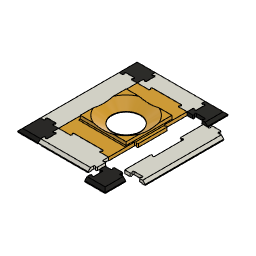
JarBase v9 (Autodesk Fusion 360 design; units mm, degrees)
Autodesk Fusion 360 part; units mm, degrees
sketch "Sketch1" plane through (0, 0, 0) normal (0, 0, 1) x (1, 0, 0) in component "JarBase"
  line L0 (32.5, -50) -> (-32.5, -50)
  line L1 (-32.5, -50) -> (-32.5, 50)
  line L2 (-32.5, 50) -> (32.5, 50)
  line L3 (32.5, 50) -> (32.5, -50)
  line L4 (32.5, -50) -> (-32.5, 50) construction
  line L5 (-32.5, -50) -> (32.5, 50) construction
  line L6 (28.5, -30) -> (-28.5, -30)
  line L7 (-28.5, -30) -> (-28.5, 30)
  line L8 (-28.5, 30) -> (28.5, 30)
  line L9 (28.5, 30) -> (28.5, -30)
  line L10 (28.5, -30) -> (-28.5, 30) construction
  line L11 (-28.5, -30) -> (28.5, 30) construction
  line L12 (28.5, 46) -> (-28.5, 46)
  line L13 (-28.5, 46) -> (-28.5, -46)
  line L14 (-28.5, -46) -> (28.5, -46)
  line L15 (28.5, -46) -> (28.5, 46)
  line L16 (28.5, 46) -> (-28.5, -46) construction
  line L17 (-28.5, 46) -> (28.5, -46) construction
  line L18 (-20, -46) -> (-16, -50)
  line L19 (-20, -46) -> (-14.5795, -46) construction
  line L20 (20, -46) -> (16, -50)
  line L21 (20, -46) -> (25.374, -46) construction
  line L22 (28.5, 16) -> (32.5, 20)
  line L23 (28.5, 16) -> (37.0214, 16) construction
  line L24 (28.5, -16) -> (32.5, -20)
  line L25 (28.5, -16) -> (34.342, -16) construction
  line L26 (-28.5, 46) -> (-32.5, 46)
  line L27 (16, 46) -> (20, 50)
  line L28 (16, 46) -> (23.4683, 46) construction
  line L29 (-16.4731, 46) -> (-20, 50)
  line L30 (-19.9118, 49.9) -> (19.9, 49.9)
  line L31 (15.8586, 46) -> (19.7586, 49.9)
  line L32 (-16.3398, 46) -> (-19.8667, 50)
  line L33 (28.5, 15.8586) -> (32.5, 19.8586)
  line L34 (32.4, 19.9) -> (32.4, -19.9)
  line L35 (32.5, -19.8586) -> (28.5, -15.8586)
  line L36 (28.5, -46) -> (28.5, -50)
  circle A0 centre (0, 0) radius 16.5
  line L37 (-55.4758, 0) -> (62.2812, 0) construction
  line L38 (-28.5, -20) -> (-32.5, -16)
  line L39 (-28.5, -20) -> (-22.6366, -20) construction
  line L40 (-28.5, 20) -> (-32.5, 16)
  line L41 (-28.5, 20) -> (-23.3061, 20) construction
  line L42 (0, 81.2463) -> (0, -111.1195) construction
  circle A1 centre (0, 0) radius 17.5
  dimension "d3" = 65
  dimension "d4" = 100
  dimension "d7" = 57
  dimension "d8" = 60
  dimension "d13" = 57
  dimension "d14" = 92
  dimension "d26" = 40
  dimension "d27" = 45
  dimension "d28" = 135
  dimension "d33" = 45
  dimension "d34" = 45
  dimension "d35" = 40
  dimension "d40" = 45
  dimension "d42" = 40
  dimension "d43" = 0.1
  dimension "d44" = 0.1
  dimension "d45" = 0.1
  dimension "d46" = 0.1
  dimension "d47" = 0.1
  dimension "d48" = 0.1
  dimension "d57" = 33
  dimension "d58" = 135
  dimension "d59" = 135
  dimension "d60" = 40
  dimension "d217" = 35
  constraint horizontal L0
  constraint perpendicular L0 L1
  constraint parallel L0 L2
  constraint parallel L1 L3
  constraint coincident L4 A0.centre
  constraint coincident L5 A0.centre
  constraint coincident A0.centre A1.centre
  constraint horizontal L6
  constraint perpendicular L6 L7
  constraint parallel L6 L8
  constraint parallel L7 L9
  constraint coincident L10 A0.centre
  constraint coincident L11 A0.centre
  constraint horizontal L12
  constraint perpendicular L12 L13
  constraint parallel L12 L14
  constraint parallel L13 L15
  constraint coincident L16 A0.centre
  constraint coincident L17 A0.centre
  constraint horizontal L19
  constraint horizontal L21
  constraint coincident L0 L20.end
  constraint horizontal L23
  constraint horizontal L25
  constraint coincident L3 L24.end
  constraint coincident L1 L26.end
  constraint perpendicular L1 L26
  constraint horizontal L28
  constraint coincident L2 L27.end
  constraint coincident L2 L29.end
  constraint coincident L14 L20.start
  constraint coincident L15 L24.start
  constraint coincident L15 L22.start
  constraint coincident L12 L27.start
  constraint coincident L12 L29.start
  constraint coincident L29 L30.start
  constraint coincident L27 L30.end
  constraint parallel L2 L30
  constraint coincident L12 L31.start
  constraint coincident L30 L31.end
  constraint parallel L27 L31
  constraint coincident L12 L32.start
  constraint coincident L2 L32.end
  constraint parallel L29 L32
  constraint coincident L15 L33.start
  constraint coincident L3 L33.end
  constraint parallel L22 L33
  constraint coincident L22 L34.start
  constraint coincident L24 L34.end
  constraint vertical L34
  constraint coincident L3 L35.start
  constraint coincident L15 L35.end
  constraint parallel L24 L35
  constraint coincident L0 L36.end
  constraint perpendicular L0 L36
  constraint coincident L0 L18.end
  constraint horizontal L37
  constraint coincident A0.centre L37
  constraint horizontal L39
  constraint coincident L1 L38.end
  constraint horizontal L41
  constraint coincident L7 L40.start
  constraint coincident L1 L40.end
  constraint symmetric L38.start L37 L40.start
  constraint coincident L3 L22.end
  constraint symmetric L22.end L24.end L37
  constraint coincident L14 L18.start
  constraint perpendicular L14 L42
  constraint coincident A0.centre L42
  constraint symmetric L18.start L20.start L42
  constraint symmetric L27.end L29.end L42
  constraint concentric A0 A1
  measures "d3" distance of L1.end L2.end
  measures "d4" distance of L0 L2
  measures "d7" distance of L7.end L8.end
  measures "d8" distance of L6.end L7.end
  measures "d13" distance of L13.end L14.end
  measures "d14" distance of L12.end L13.end
  measures "d26" distance of L18.start L20.start
  measures "d27" angle of L18 L19
  measures "d28" angle of L20 L21
  measures "d33" angle of L22 L23
  measures "d34" angle of L24 L25
  measures "d35" vertical distance of L22.end L24.end
  measures "d40" angle of L27 L28
  measures "d42" distance of L27.end L29.end
  measures "d43" distance of L2 L30
  measures "d44" distance of L27 L31
  measures "d45" distance of L29 L32
  measures "d46" distance of L22 L33
  measures "d47" distance of L3 L34
  measures "d48" distance of L24 L35
  measures "d57" diameter of A0
  measures "d58" angle of L38 L39
  measures "d59" angle of L40 L41
  measures "d60" distance of L38.start L40.start
  measures "d217" diameter of A1
extrude "Extrude1" add sketch "Sketch1" along normal blind 4 contours L0 L14 L20 L36 | L6 L13 L14 L15 | L0 L1 L7 L13 L14 L18 L38 | L6 L7 L8 L9 L13 L15 | L9 L15 L33 L34 L35 | L1 L7 L13 L26 L40 | L8 L12 L13 L15 | L12 L30 L31 L32 | A0 | A1 makes body 1 in component "JarBase"
sketch "Sketch5" plane through (0, 0, 4) normal (0, 0, 1) x (-1, 0, 0) in component "JarBase"
  line L0 (-28.5, -15.8586) -> (-28.5, -46)
  line L1 (-28.5, -46) -> (-15.8586, -46)
  line L2 (-15.8586, -46) -> (-19.7586, -49.9)
  line L3 (-19.7586, -49.9) -> (19.7785, -49.9)
  line L4 (19.7785, -49.9) -> (16.3398, -46)
  line L5 (16.3398, -46) -> (32.5, -46)
  line L6 (32.5, -46) -> (32.5, -16)
  line L7 (32.5, 50) -> (16, 50)
  line L8 (16, 50) -> (20, 46)
  line L9 (20, 46) -> (-20, 46)
  line L10 (-28.5, 15.8586) -> (-32.4, 19.7586)
  line L11 (-32.4, 19.7586) -> (-32.4, -19.7586)
  line L12 (-32.4, -19.7586) -> (-28.5, -15.8586)
  line L13 (28, -28) -> (-28, -28)
  line L14 (-28, -28) -> (-28, 28)
  line L15 (-28, 28) -> (28, 28)
  line L16 (28, 28) -> (28, -28)
  line L17 (28, -28) -> (-28, 28) construction
  line L18 (-28, -28) -> (28, 28) construction
  line L19 (32.5, -16) -> (28.5, -20)
  line L20 (28.5, -20) -> (28.5, 20)
  line L21 (28.5, 20) -> (32.5, 16)
  line L22 (32.5, 16) -> (32.5, 50)
  line L23 (-20, 46) -> (-16, 50)
  line L24 (-16, 50) -> (-28.5, 50)
  line L25 (-28.5, 50) -> (-28.5, 15.8586)
  dimension "d51" = 56
  dimension "d52" = 56
  constraint horizontal L13
  constraint perpendicular L13 L14
  constraint parallel L13 L15
  constraint parallel L14 L16
  constraint coincident L17 origin
  constraint coincident L18 origin
  measures "d51" distance of L14.end L15.end
  measures "d52" distance of L13.end L14.end
extrude "Extrude3" add sketch "Sketch5" along normal blind 5 contours L13 L14 L15 L16 bodies 1 in component "JarBase"
sketch "Sketch3" plane through (0, 0, 9) normal (0, 0, 1) x (-1, 0, 0) in component "JarBase"
  circle A0 centre (0, 0) radius 30.5
  line L0 (30, 30) -> (-30, 30)
  line L1 (-30, 30) -> (-30, -30)
  line L2 (-30, -30) -> (30, -30)
  line L3 (30, -30) -> (30, 30)
  line L4 (28, 28) -> (-28, 28)
  line L5 (-28, 28) -> (-28, -28)
  line L6 (-28, -28) -> (28, -28)
  line L7 (28, -28) -> (28, 28)
  dimension "d12" = 61
  constraint coincident A0.centre origin
  measures "d12" diameter of A0
fillet "Fillet1" radius 1 16 edges at (-19.7785, 49.9, 2) (-16.3398, 46, 2) (19.7586, 49.9, 2) (15.8586, 46, 2) (32.4, 19.7586, 2) (32.4, -19.7586, 2) (28.5, -15.8586, 2) (28.5, 15.8586, 2) (20, -46, 2) (16, -50, 2) (-16, -50, 2) (-20, -46, 2) (-32.5, -16, 2) (-28.5, -20, 2) (-32.5, 16, 2) (-28.5, 20, 2) on bodies 1 in component "JarBase"
loft "Loft2" cut profiles "Sketch1", "Sketch3" section 1 contours A0 section 2 contours A0 L3 | A0 L3 L7 | A0 L4 L5 L6 L7 | A0 L0 L4 | A0 L0 | A0 L2 L6 | A0 L2 | A0 L1 L5 | A0 L1 bodies 1 in component "JarBase"
fillet "Fillet2" radius 1 4 edges at (0, 28, 4) (-28, 0, 4) (0, -28, 4) (28, 0, 4) on bodies 1 in component "JarBase"
sketch "Sketch1 (2)" plane through (0, 0, 0) normal (0, 0, 1) x (1, 0, 0) in component "TopEdge"
  line L0 (28.5, 46) -> (28.5, 71)
  line L1 (28.5, 71) -> (-32.5, 71)
  line L2 (-32.5, 71) -> (-32.5, 46)
  line L3 (-32.5, 52) -> (28.5, 52)
  line L4 (-32.5, 67) -> (28.5, 67)
  line L5 (-32.5, 50) -> (32.5, 50)
  line L6 (16, 46) -> (20, 50)
  line L7 (16, 46) -> (23.4683, 46)
  line L8 (28.5, 46) -> (-28.5, 46)
  line L9 (-16.4731, 46) -> (-20, 50)
  line L10 (-32.5, 46) -> (28.5, 46)
  line L11 (-20, 50) -> (-16.4731, 46)
  line L12 (20, 50) -> (16, 46)
  line L13 (20, 50) -> (-20, 50)
  line L14 (-28.5, 71) -> (-28.5, 46)
  line L15 (32.5, 66) -> (32.5, 51)
  line L16 (-32.5, 62) -> (-28.5, 66)
  line L17 (-32.5, 62) -> (-26.8431, 62) construction
  line L18 (-32.5, 55) -> (-28.5, 51)
  line L19 (-51.9513, 58.5) -> (44.591, 58.5) construction
  line L20 (32.5, 51) -> (28.5, 55)
  line L21 (32.5, 51) -> (38.1569, 51) construction
  line L22 (32.5, 66) -> (28.5, 62)
  line L23 (28.5, 61.8586) -> (32.4, 65.7586)
  line L24 (28.5, 55.1414) -> (32.5, 51.1414)
  line L25 (32.4, 65.7586) -> (32.4, 51.2414)
  point P0 (-32.5, 46)
  dimension "d62" = 15
  dimension "d63" = 4
  dimension "d64" = 25
  dimension "d81" = 4
  dimension "d82" = 4
  dimension "d83" = 45
  dimension "d84" = 90
  dimension "d85" = 15
  dimension "d86" = 135
  dimension "d87" = 90
  dimension "d88" = 15
  dimension "d89" = 0.1
  dimension "d90" = 0.1
  dimension "d91" = 0.1
  constraint vertical L0
  constraint horizontal L1
  constraint vertical L2
  constraint coincident L2 L3.start
  constraint coincident L0 L3.end
  constraint perpendicular L0 L3
  constraint coincident L2 L4.start
  constraint coincident L0 L4.end
  constraint perpendicular L0 L4
  constraint coincident L0.start L8.start
  constraint perpendicular L0 L10
  constraint coincident L9.end L11.start
  constraint coincident L9.start L11.end
  constraint coincident L6.end L12.start
  constraint coincident L6.start L7.start
  constraint coincident L0 L8.start
  constraint coincident L2 P0
  constraint coincident L1 L14.start
  constraint coincident L10 L8.end
  constraint perpendicular L10 L14
  constraint vertical L15
  constraint horizontal L17
  constraint coincident L2 L16.start
  constraint coincident L14 L16.end
  constraint coincident L2 L18.start
  constraint coincident L14 L18.end
  constraint horizontal L19
  constraint symmetric L1 L10 L19
  constraint symmetric L16.end L18.end L19
  constraint symmetric L15.start L15.end L19
  constraint horizontal L21
  constraint coincident L0 L20.end
  constraint coincident L0 L22.end
  constraint coincident L0 L23.start
  constraint parallel L22 L23
  constraint coincident L0 L24.start
  constraint coincident L15 L24.end
  constraint perpendicular L23 L24
  constraint coincident L23 L25.start
  constraint coincident L24 L25.end
  constraint parallel L15 L25
  constraint coincident L23.end L25
  measures "d62" distance of L3 L4
  measures "d63" distance of L1 L4
  measures "d64" distance of L1 L10
  measures "d81" distance of L2 L14
  measures "d82" distance of L0 L15
  measures "d83" angle of L16 L17
  measures "d84" angle of L16 L18
  measures "d85" distance of L16.end L18.end
  measures "d86" angle of L20 L21
  measures "d87" angle of L20 L22
  measures "d88" distance of L15.start L15.end
  measures "d89" distance of L22 L23
  measures "d90" distance of L20 L24
  measures "d91" distance of L15 L25
extrude "Extrude1'" add sketch "Sketch1 (2)" along normal blind 4 separate body contours L0 L3 L4 L14 | L0 L3 L5 L13 L14 | L0 L5 L6 L7 L8 L10 L12 | L0 L23 L24 L25 | L2 L3 L5 L14 L18 | L2 L3 L18 | L2 L4 L14 L16 | L5 L8 L9 L10 L11 L14 | L0 L1 L4 L14 | L1 L2 L4 L14 | L2 L5 L10 L14 makes body 2 in component "TopEdge"
fillet "Fillet1'" radius 1 4 edges at (-16.4731, 46, 2) (-20, 50, 2) (20, 50, 2) (16, 46, 2) on bodies 2 in component "TopEdge"
extrude "Extrude2" cut sketch "Sketch1 (2)" along normal blind 0.5 contours L0 L3 L4 L14 | L2 L3 L14 L16 L18 | L0 L23 L24 L25 | L2 L3 L18 | L2 L4 L14 L16 bodies 2 in component "TopEdge"
sketch "Sketch1 (3)" plane through (0, 0, 0) normal (0, 0, 1) x (1, 0, 0) in component "RIghtEdge"
  line L0 (28.5, 46) -> (53.5, 46)
  line L1 (53.5, 46) -> (53.5, -50)
  line L2 (53.5, -50) -> (28.5, -50)
  line L3 (28.5, -50) -> (28.5, 46)
  line L4 (28.5, 16) -> (32.5, 20)
  line L5 (32.5, 50) -> (32.5, -50)
  line L6 (28.5, -16) -> (32.5, -20)
  line L7 (28.5, 16) -> (32.5, 20)
  line L8 (32.5, -20) -> (28.5, -16)
  line L9 (32.5, 20) -> (32.5, -20)
  line L10 (49.5, 46) -> (49.5, -50)
  line L11 (34.5, 46) -> (34.5, -50)
  line L12 (41, 52.9761) -> (41, -53.7829) construction
  line L13 (29.9594, 46) -> (43.3433, 46) construction
  line L14 (48.5, 50) -> (44.5, 46)
  line L15 (48.5, 50) -> (48.5481, 50) construction
  line L16 (33.5, 50) -> (37.6148, 45.8852)
  line L17 (33.5, 50) -> (39.2756, 50) construction
  line L18 (33.5, 50) -> (48.5, 50)
  line L19 (33.6414, 50) -> (37.6414, 46)
  line L20 (48.3586, 50) -> (44.3586, 46)
  line L21 (33.7414, 49.9) -> (48.2586, 49.9)
  line L22 (33.5, -46) -> (48.5, -46)
  line L23 (48.5, -46) -> (44.5, -50)
  line L24 (48.5, -46) -> (54.0005, -46) construction
  line L25 (33.5, -46) -> (37.5, -50)
  point P0 (28.5, 46)
  dimension "d71" = 96
  dimension "d72" = 25
  dimension "d73" = 4
  dimension "d74" = 15
  dimension "d119" = 135
  dimension "d120" = 45
  dimension "d121" = 15
  dimension "d122" = 4
  dimension "d123" = 0.1
  dimension "d124" = 0.1
  dimension "d125" = 0.1
  dimension "d126" = 15
  dimension "d127" = 4
  dimension "d128" = 135
  dimension "d129" = 90
  constraint horizontal L0
  constraint vertical L1
  constraint horizontal L2
  constraint vertical L3
  constraint coincident P0 L0.start
  constraint coincident L4.start L7.start
  constraint coincident L4.end L7.end
  constraint coincident L6.end L8.start
  constraint coincident L6.start L8.end
  constraint coincident L0 L10.start
  constraint coincident L2 L10.end
  constraint perpendicular L2 L10
  constraint coincident L0 L11.start
  constraint coincident L2 L11.end
  constraint perpendicular L2 L11
  constraint perpendicular L0 L12
  constraint horizontal L13
  constraint coincident L0 L13.start
  constraint horizontal L15
  constraint horizontal L17
  constraint coincident L0 L14.end
  constraint symmetric L12 L14.start L16.start
  constraint coincident L18 L19.start
  constraint coincident L13 L19.end
  constraint coincident L18 L20.start
  constraint coincident L0 L20.end
  constraint perpendicular L19 L20
  constraint coincident L19 L21.start
  constraint coincident L20 L21.end
  constraint horizontal L21
  constraint parallel L16 L19
  constraint perpendicular L12 L22
  constraint horizontal L24
  constraint coincident L2 L23.end
  constraint coincident L2 L25.end
  constraint symmetric L12 L23 L25
  measures "d71" distance of L0.end L2
  measures "d72" distance of L1 L3
  measures "d73" distance of L1 L10
  measures "d74" distance of L10 L11
  measures "d119" angle of L14 L15
  measures "d120" angle of L16 L17
  measures "d121" distance of L14.start L16.start
  measures "d122" distance of L0 L18
  measures "d123" distance of L18 L21
  measures "d124" distance of L14 L20
  measures "d125" distance of L16 L19
  measures "d126" distance of L22.start L22.end
  measures "d127" distance of L2 L22
  measures "d128" angle of L23 L24
  measures "d129" angle of L23 L25
extrude "Extrude1''" add sketch "Sketch1 (3)" along normal blind 4 separate body contours L0 L19 L20 L21 | L0 L2 L10 L11 L22 L23 | L0 L2 L5 L9 L11 L22 L25 | L0 L1 L2 L10 | L0 L3 L4 L5 L7 | L2 L11 L25 | L2 L3 L5 L6 L8 makes body 3 in component "RIghtEdge"
extrude "Extrude2'" cut sketch "Sketch1 (3)" along normal blind 0.5 contours L0 L19 L20 L21 | L0 L2 L10 L11 L22 L23 | L2 L11 L22 L23 L25 | L2 L11 L25 bodies 3 in component "RIghtEdge"
fillet "Fillet1''" radius 1 4 edges at (28.5, 16, 2) (32.5, 20, 2) (28.5, -16, 2) (32.5, -20, 2) on bodies 3 in component "RIghtEdge"
fillet "Fillet2'" radius 1 4 edges at (-28.5, 66, 2.25) (-32.5, 62, 2.25) (-28.5, 51, 2) (-32.5, 55, 2.25) on bodies 2 in component "TopEdge"
fillet "Fillet3" radius 1 4 edges at (28.5, 61.8586, 2.25) (32.4, 65.7586, 2) (32.4, 51.2414, 2) (28.5, 55.1414, 2.25) on bodies 2 in component "TopEdge"
sketch "Sketch1 (4)" plane through (0, 0, 0) normal (0, 0, 1) x (1, 0, 0) in component "TopRightCorner"
  line L0 (32.5, 66) -> (28.5, 62)
  line L1 (32.5, 66) -> (32.5, 51)
  line L2 (32.5, 51) -> (28.5, 55)
  line L3 (28.5, 46) -> (28.5, 71)
  line L4 (28.5, 46) -> (53.5, 46)
  line L5 (28.5, 71) -> (53.5, 71)
  line L6 (53.5, 71) -> (53.5, 46)
  line L7 (53.5, 46) -> (28.5, 46)
  line L8 (28.5, 46) -> (28.5, 71)
  line L9 (32.5, 66) -> (28.5, 62)
  line L10 (28.5, 62) -> (28.5, 71)
  line L11 (32.5, 66) -> (32.5, 51)
  line L12 (32.5, 51) -> (28.5, 55)
  line L13 (28.5, 55) -> (28.5, 46)
  line L14 (28.5, 46) -> (37.5, 46)
  line L15 (44.5, 46) -> (53.5, 46)
  line L16 (33.5, 50) -> (48.5, 50)
  line L17 (33.5, 50) -> (37.6148, 45.8852)
  line L18 (48.5, 50) -> (44.5, 46)
  line L19 (53.5, 46) -> (44.3586, 46)
  line L20 (29.9594, 46) -> (43.3433, 46)
  line L21 (28.5, 46) -> (37.5, 46)
  line L22 (37.5, 46) -> (33.5, 50)
  line L23 (33.5, 50) -> (48.5, 50)
  line L24 (48.5, 50) -> (44.5, 46)
  line L25 (44.5, 46) -> (53.5, 46)
  point P0 (43.3433, 46)
  constraint horizontal L5
  constraint vertical L6
  constraint horizontal L7
  constraint vertical L8
  constraint coincident L4.end L6.end
  constraint coincident L3.end L5.start
  constraint coincident L0.start L1.start
  constraint coincident L0.end L9.end
  constraint coincident L1.end L2.start
  constraint coincident L2.end L12.end
  constraint coincident L3.start L4.start
  constraint parallel L20 L21
  constraint coincident L16.start L17.start
  constraint parallel L17 L22
  constraint coincident L16.end L18.start
  constraint parallel L18 L24
  constraint perpendicular L6 L25
extrude "Extrude1'''" add sketch "Sketch1 (4)" along normal blind 4 separate body contours L0 L1 L2 L3 L4 L5 L6 L7 L8 L9 L10 L11 L12 L13 L14 L15 L16 L17 L18 L19 L20 L21 L22 L23 L24 L25 makes body 4 in component "TopRightCorner"
fillet "Fillet1'''" radius 1 8 edges at (32.5, 51, 2) (28.5, 55, 2) (32.5, 66, 2) (28.5, 62, 2) (33.5, 50, 2) (37.5, 46, 2) (48.5, 50, 2) (44.5, 46, 2) on bodies 4 in component "TopRightCorner"
chamfer "Chamfer1" distance 3 angle 45 2 edges at (53.5, 58.5, 4) (41, 71, 4) on bodies 4 in component "TopRightCorner"
chamfer "Chamfer1'" distance 3 angle 45 1 edges at (53.5, -2, 4) on bodies 3 in component "RIghtEdge"
chamfer "Chamfer1''" distance 3 angle 45 1 edges at (-2, 71, 4) on bodies 2 in component "TopEdge"
fillet "Fillet3'" radius 1 8 edges at (37.6414, 46, 2.25) (33.7414, 49.9, 2.25) (48.2586, 49.9, 2.25) (44.3586, 46, 2.25) (37.5, -50, 2.25) (33.5, -46, 2) (48.5, -46, 2.25) (44.5, -50, 2.25) on bodies 3 in component "RIghtEdge"
sketch "Sketch1 (5)" plane through (0, 0, 0) normal (0, 0, 1) x (1, 0, 0) in component "BottomEdge"
  line L0 (32.5, -50) -> (-32.5, -50)
  line L1 (-20, -46) -> (-16, -50)
  line L2 (-28.5, -46) -> (28.5, -46)
  line L3 (20, -46) -> (16, -50)
  line L4 (28.5, -46) -> (28.5, -50)
  line L5 (-32.5, -50) -> (28.5, -50)
  line L6 (28.5, -50) -> (28.5, -75)
  line L7 (28.5, -75) -> (-32.5, -75)
  line L8 (-32.5, -75) -> (-32.5, -50)
  line L9 (-32.5, -50) -> (-16, -50)
  line L10 (-16, -50) -> (-20, -46)
  line L11 (-20, -46) -> (20, -46)
  line L12 (20, -46) -> (16, -50)
  line L13 (16, -50) -> (28.5, -50)
  line L14 (-19.8586, -46) -> (-15.8586, -50)
  line L15 (19.8586, -46) -> (15.8586, -50)
  line L16 (-19.7586, -46.1) -> (19.7586, -46.1)
  line L17 (32.5, -55) -> (32.5, -70)
  line L18 (-44.7263, -62.5) -> (51.0183, -62.5) construction
  line L19 (32.5, -55) -> (28.5, -59)
  line L20 (32.5, -55) -> (26.9554, -55) construction
  line L21 (32.5, -70) -> (28.5, -66)
  line L22 (32.5, -70) -> (26.9554, -70) construction
  line L23 (32.5, -55.1414) -> (28.5, -59.1414)
  line L24 (28.5, -65.8586) -> (32.5, -69.8586)
  line L25 (32.4, -55.2414) -> (32.4, -69.7586)
  line L26 (28.5, -56) -> (-32.5, -56)
  line L27 (28.5, -71) -> (-32.5, -71)
  line L28 (-28.5, -50) -> (-28.5, -75)
  line L29 (-28.5, -56) -> (-19.8335, -56) construction
  line L30 (-28.5, -55) -> (-32.5, -59)
  line L31 (-28.5, -55) -> (-22.8431, -55) construction
  line L32 (-28.5, -70) -> (-32.5, -66)
  dimension "d133" = 0.1
  dimension "d134" = 0.1
  dimension "d135" = 0.1
  dimension "d136" = 15
  dimension "d137" = 45
  dimension "d138" = 45
  dimension "d139" = 0.1
  dimension "d140" = 0.1
  dimension "d141" = 0.1
  dimension "d142" = 4
  dimension "d143" = 15
  dimension "d146" = 4
  dimension "d148" = 4
  dimension "d149" = 135
  dimension "d150" = 90
  dimension "d151" = 15
  dimension "d167" = 25
  constraint horizontal L5
  constraint vertical L6
  constraint horizontal L7
  constraint vertical L8
  constraint coincident L0.end L5.start
  constraint coincident L4.end L6
  constraint coincident L1.end L9.end
  constraint coincident L1.start L10.end
  constraint coincident L3.start L11.end
  constraint coincident L3.end L12.end
  constraint coincident L4.end L5.end
  constraint coincident L11 L14.start
  constraint coincident L0 L14.end
  constraint coincident L2 L15.start
  constraint coincident L0 L15.end
  constraint coincident L14 L16.start
  constraint coincident L15 L16.end
  constraint parallel L13 L16
  constraint parallel L1 L14
  constraint parallel L12 L15
  constraint vertical L17
  constraint horizontal L18
  constraint symmetric L5 L7 L18
  constraint symmetric L17.start L17.end L18
  constraint horizontal L20
  constraint coincident L6 L19.end
  constraint horizontal L22
  constraint coincident L6 L21.end
  constraint coincident L17 L23.start
  constraint parallel L19 L23
  constraint coincident L6 L24.start
  constraint coincident L17 L24.end
  constraint perpendicular L23 L24
  constraint coincident L23 L25.start
  constraint coincident L24 L25.end
  constraint perpendicular L18 L25
  constraint coincident L6 L26.start
  constraint coincident L8 L26.end
  constraint perpendicular L8 L26
  constraint coincident L6 L27.start
  constraint coincident L8 L27.end
  constraint perpendicular L8 L27
  constraint coincident L9 L28.start
  constraint coincident L7 L28.end
  constraint perpendicular L7 L28
  constraint horizontal L29
  constraint coincident L28 L29.start
  constraint coincident L26 L29.start
  constraint horizontal L31
  constraint coincident L28 L30.start
  constraint coincident L8 L30.end
  constraint coincident L28 L32.start
  constraint coincident L8 L32.end
  constraint symmetric L18 L30.start L32.start
  constraint coincident L6 L23.end
  measures "d133" distance of L10 L14
  measures "d134" distance of L3 L15
  measures "d135" distance of L11 L16
  measures "d136" distance of L17.start L17.end
  measures "d137" angle of L19 L20
  measures "d138" angle of L21 L22
  measures "d139" distance of L19 L23
  measures "d140" distance of L17 L25
  measures "d141" distance of L21 L24
  measures "d142" distance of L6 L17
  measures "d143" distance of L26 L27
  measures "d146" distance of L8 L28
  measures "d148" distance of L7 L27
  measures "d149" angle of L30 L31
  measures "d150" angle of L30 L32
  measures "d151" distance of L30.start L32.start
  measures "d167" distance of L0 L7
extrude "Extrude1''''" add sketch "Sketch1 (5)" along normal blind 4 separate body contours L0 L5 L6 L9 L13 L26 L28 | L6 L26 L27 L28 | L0 L5 L14 L15 L16 | L6 L23 L24 L25 | L8 L26 L30 | L0 L5 L8 L9 L26 L28 L30 | L8 L27 L28 L32 | L7 L8 L27 L28 | L6 L7 L27 L28 makes body 5 in component "BottomEdge"
extrude "Extrude2''" cut sketch "Sketch1 (5)" along normal blind 0.5 contours L0 L5 L6 L9 L13 L26 L28 | L6 L26 L27 L28 | L8 L26 L28 L30 L32 | L26 L28 L30 | L6 L23 L24 L25 | L8 L26 L30 | L0 L5 L8 L9 L26 L28 L30 | L8 L27 L28 L32 | L7 L8 L27 L28 bodies 5 in component "BottomEdge"
chamfer "Chamfer1'''" distance 3 angle 45 1 edges at (-2, -75, 4) on bodies 5 in component "BottomEdge"
sketch "Sketch1 (6)" plane through (0, 0, 0) normal (0, 0, 1) x (1, 0, 0) in component "RightBottomCorner"
  line L0 (53.5, -50) -> (28.5, -50)
  line L1 (33.5, -46) -> (48.5, -46)
  line L2 (33.5, -46) -> (37.5, -50)
  line L3 (48.5, -46) -> (44.5, -50)
  line L4 (28.5, -50) -> (28.5, -75)
  line L5 (32.5, -55) -> (28.5, -59)
  line L6 (32.5, -55) -> (32.5, -70)
  line L7 (32.5, -70) -> (28.5, -66)
  line L8 (28.5, -50) -> (53.5, -50)
  line L9 (53.5, -50) -> (53.5, -75)
  line L10 (53.5, -75) -> (28.5, -75)
  line L11 (28.5, -75) -> (28.5, -50)
  line L12 (28.5, -59) -> (32.5, -55)
  line L13 (32.5, -55) -> (32.5, -70)
  line L14 (32.5, -70) -> (27.5, -65)
  line L15 (37.5, -50) -> (33.5, -46)
  line L16 (33.5, -46) -> (48.5, -46)
  line L17 (48.5, -46) -> (44.5, -50)
  line L18 (33.6414, -46) -> (37.6414, -50)
  line L19 (48.3586, -46) -> (44.3586, -50)
  line L20 (33.7414, -46.1) -> (48.2586, -46.1)
  point P0 (53.5, -50)
  dimension "d159" = 0.1
  dimension "d160" = 0.1
  dimension "d161" = 0.1
  constraint horizontal L8
  constraint vertical L9
  constraint horizontal L10
  constraint vertical L11
  constraint coincident L0.end L4.start
  constraint coincident L9 P0
  constraint coincident L4.end L10
  constraint coincident L5.end L12.start
  constraint coincident L5.start L6.start
  constraint coincident L6.end L7.start
  constraint parallel L7 L14
  constraint coincident L2.end L15.start
  constraint coincident L1.start L2.start
  constraint coincident L1.end L3.start
  constraint coincident L3.end L17.end
  constraint coincident L1 L18.start
  constraint coincident L0 L18.end
  constraint parallel L15 L18
  constraint coincident L16 L19.start
  constraint coincident L8 L19.end
  constraint perpendicular L18 L19
  constraint coincident L18 L20.start
  constraint coincident L19 L20.end
  constraint parallel L1 L20
  measures "d159" distance of L15 L18
  measures "d160" distance of L16 L20
  measures "d161" distance of L17 L19
extrude "Extrude1'''''" add sketch "Sketch1 (6)" along normal blind 4 separate body contours L0 L4 L5 L6 L7 L8 L9 L10 L11 L12 L13 L14 | L0 L8 L18 L19 L20 makes body 6 in component "RightBottomCorner"
fillet "Fillet1''''" radius 1 8 edges at (28.5, -59, 2) (32.5, -55, 2) (32.5, -70, 2) (28.5, -66, 2) (37.6414, -50, 2) (33.7414, -46.1, 2) (48.2586, -46.1, 2) (44.3586, -50, 2) on bodies 6 in component "RightBottomCorner"
chamfer "Chamfer1''''" distance 3 angle 45 2 edges at (53.5, -62.5, 4) (41, -75, 4) on bodies 6 in component "RightBottomCorner"
sketch "Sketch1 (7)" plane through (0, 0, 0) normal (0, 0, 1) x (1, 0, 0) in component "LeftEdge"
  line L0 (-32.5, -50) -> (-32.5, 50)
  line L1 (-28.5, 20) -> (-32.5, 16)
  line L2 (-28.5, 46) -> (-28.5, -46)
  line L3 (-28.5, -20) -> (-32.5, -16)
  line L4 (-28.5, 46) -> (-32.5, 46)
  line L5 (-32.5, 46) -> (-57.5, 46)
  line L6 (-57.5, 46) -> (-57.5, -50)
  line L7 (-57.5, -50) -> (-32.5, -50)
  line L8 (-32.5, -50) -> (-32.5, 46)
  line L9 (-32.5, -46) -> (-57.5, -46)
  line L10 (-37.5, 50) -> (-52.5, 50)
  line L11 (-45, 57.6905) -> (-45, -60.3769) construction
  line L12 (-37.5, 50) -> (-41.5, 46)
  line L13 (-37.5, 50) -> (-31.8431, 50) construction
  line L14 (-52.5, 50) -> (-48.5, 46)
  line L15 (-52.5, -46) -> (-48.5, -50)
  line L16 (-52.5, -46) -> (-46.2445, -46) construction
  line L17 (-37.5, -46) -> (-41.5, -50)
  line L18 (-37.5, -46) -> (-30.9999, -46) construction
  line L19 (-52.3586, 50) -> (-48.3586, 46)
  line L20 (-37.6414, 50) -> (-41.6414, 46)
  line L21 (-52.2586, 49.9) -> (-37.7414, 49.9)
  line L22 (-53.5, 46) -> (-53.5, -50)
  line L23 (-38.5, 46) -> (-38.5, -50)
  line L24 (-32.5, 15.8586) -> (-28.5, 19.8586)
  line L25 (-32.5, -15.8586) -> (-28.5, -19.8586)
  line L26 (-28.6, 19.7586) -> (-28.6, -19.7586)
  line L27 (-28.5, -30) -> (-28.5, 30)
  point P0 (-32.5, -50)
  point P1 (-44.7263, -62.5)
  dimension "d168" = 25
  dimension "d169" = 15
  dimension "d170" = 4
  dimension "d171" = 4
  dimension "d172" = 135
  dimension "d174" = 45
  dimension "d175" = 135
  dimension "d176" = 15
  dimension "d177" = 0.1
  dimension "d178" = 0.1
  dimension "d179" = 0.1
  dimension "d180" = 4
  dimension "d181" = 15
  dimension "d182" = 0.1
  dimension "d183" = 0.1
  dimension "d184" = 0.1
  constraint horizontal L5
  constraint vertical L6
  constraint horizontal L7
  constraint vertical L8
  constraint coincident L4.end L5.start
  constraint coincident L7 P0
  constraint coincident L8 L9.start
  constraint coincident L6 L9.end
  constraint perpendicular L6 L9
  constraint perpendicular L0 L10
  constraint vertical L11
  constraint symmetric L6 L8 L11
  constraint symmetric L10.start L10.end L11
  constraint horizontal L13
  constraint coincident L5 L12.end
  constraint coincident L5 L14.end
  constraint perpendicular L12 L14
  constraint horizontal L16
  constraint coincident L9 L15.start
  constraint coincident L7 L15.end
  constraint horizontal L18
  constraint coincident L9 L17.start
  constraint coincident L7 L17.end
  constraint symmetric L11 L15.start L17.start
  constraint coincident L10 L19.start
  constraint coincident L5 L19.end
  constraint parallel L14 L19
  constraint coincident L10 L20.start
  constraint coincident L5 L20.end
  constraint coincident L19 L21.start
  constraint coincident L20 L21.end
  constraint perpendicular L11 L21
  constraint parallel L12 L20
  constraint coincident L5 L22.start
  constraint coincident L7 L22.end
  constraint perpendicular L7 L22
  constraint coincident L5 L23.start
  constraint coincident L7 L23.end
  constraint perpendicular L7 L23
  constraint coincident L8 L24.start
  constraint coincident L2 L24.end
  constraint coincident L0 L25.start
  constraint coincident L2 L25.end
  constraint coincident L24 L26.start
  constraint coincident L25 L26.end
  constraint parallel L2 L26
  constraint parallel L1 L24
  constraint parallel L3 L25
  measures "d168" distance of L6 L8
  measures "d169" distance of L10.start L10.end
  measures "d170" distance of L7 L9
  measures "d171" distance of L5 L10
  measures "d172" angle of L12 L13
  measures "d174" angle of L15 L16
  measures "d175" angle of L17 L18
  measures "d176" distance of L15.start L17.start
  measures "d177" distance of L14 L19
  measures "d178" distance of L12 L20
  measures "d179" distance of L10 L21
  measures "d180" distance of L6 L22
  measures "d181" distance of L22 L23
  measures "d182" distance of L1 L24
  measures "d183" distance of L26 L27
  measures "d184" distance of L3 L25
extrude "Extrude1''''''" add sketch "Sketch1 (7)" along normal blind 4 separate body contours L0 L7 L8 L9 L17 L23 | L0 L5 L8 L9 L23 | L7 L17 L23 | L0 L8 L24 L25 L26 | L5 L9 L22 L23 | L7 L9 L15 L22 | L6 L7 L9 L22 | L5 L6 L9 L22 | L5 L19 L20 L21 makes body 7 in component "LeftEdge"
extrude "Extrude2'''" cut sketch "Sketch1 (7)" along normal blind 0.5 contours L7 L17 L23 | L5 L9 L22 L23 | L7 L9 L15 L22 | L5 L19 L20 L21 bodies 7 in component "LeftEdge"
fillet "Fillet1'''''" radius 1 12 edges at (-52.5, -46, 2.25) (-48.5, -50, 2.25) (-37.5, -46, 2) (-41.5, -50, 2.25) (-28.6, -19.7586, 2) (-28.6, 19.7586, 2) (-32.5, 15.8586, 2) (-32.5, -15.8586, 2) (-48.3586, 46, 2.25) (-37.7414, 49.9, 2.25) (-52.2586, 49.9, 2.25) (-41.6414, 46, 2.25) on bodies 7 in component "LeftEdge"
chamfer "Chamfer1'''''" distance 3 angle 45 1 edges at (-57.5, -2, 4) on bodies 7 in component "LeftEdge"
sketch "Sketch1 (8)" plane through (0, 0, 0) normal (0, 0, 1) x (1, 0, 0) in component "BottomLeftCorner"
  line L0 (-57.5, -50) -> (-32.5, -50)
  line L1 (-52.5, -46) -> (-48.5, -50)
  line L2 (-32.5, -46) -> (-57.5, -46)
  line L3 (-37.5, -46) -> (-41.5, -50)
  line L4 (-32.5, -75) -> (-32.5, -50)
  line L5 (-28.5, -55) -> (-32.5, -59)
  line L6 (-28.5, -50) -> (-28.5, -75)
  line L7 (-28.5, -70) -> (-32.5, -66)
  line L8 (-57.5, -50) -> (-32.5, -50)
  line L9 (-32.5, -50) -> (-32.5, -75)
  line L10 (-32.5, -75) -> (-57.5, -75)
  line L11 (-57.5, -75) -> (-57.5, -50)
  line L12 (-52.5, -46) -> (-48.5, -50)
  line L13 (-52.5, -46) -> (-37.5, -46)
  line L14 (-37.5, -46) -> (-41.5, -50)
  line L15 (-28.5, -55) -> (-32.5, -59)
  line L16 (-28.5, -55) -> (-28.5, -70)
  line L17 (-28.5, -70) -> (-32.5, -66)
  line L18 (-52.3586, -46) -> (-48.3586, -50)
  line L19 (-37.6414, -46) -> (-41.6414, -50)
  line L20 (-52.2586, -46.1) -> (-37.7414, -46.1)
  line L21 (-32.5, -59.1414) -> (-28.5, -55.1414)
  line L22 (-32.5, -65.8586) -> (-28.5, -69.8586)
  line L23 (-28.6, -55.2414) -> (-28.6, -69.7586)
  dimension "d192" = 0.1
  dimension "d193" = 0.1
  dimension "d194" = 0.1
  dimension "d195" = 0.1
  dimension "d196" = 0.1
  dimension "d197" = 0.1
  constraint horizontal L8
  constraint vertical L9
  constraint horizontal L10
  constraint vertical L11
  constraint coincident L4.start L9.end
  constraint coincident L0.start L8.start
  constraint coincident L1.start L12.start
  constraint coincident L1.end L12.end
  constraint coincident L3.start L13.end
  constraint coincident L3.end L14.end
  constraint coincident L5.start L15.start
  constraint coincident L5.end L15.end
  constraint coincident L7.start L16.end
  constraint coincident L7.end L17.end
  constraint coincident L2 L18.start
  constraint coincident L8 L18.end
  constraint parallel L17 L18
  constraint coincident L13 L19.start
  constraint coincident L8 L19.end
  constraint perpendicular L18 L19
  constraint coincident L18 L20.start
  constraint coincident L19 L20.end
  constraint parallel L13 L20
  constraint coincident L9 L21.start
  constraint coincident L16 L21.end
  constraint coincident L4 L22.start
  constraint coincident L16 L22.end
  constraint coincident L21 L23.start
  constraint coincident L22 L23.end
  constraint vertical L23
  constraint parallel L5 L21
  constraint parallel L7 L22
  measures "d192" distance of L12 L18
  measures "d193" distance of L2 L20
  measures "d194" distance of L14 L19
  measures "d195" distance of L5 L21
  measures "d196" distance of L7 L22
  measures "d197" distance of L16 L23
extrude "Extrude1'''''''" add sketch "Sketch1 (8)" along normal blind 4 separate body contours L0 L4 L8 L9 L10 L11 | L0 L8 L18 L19 L20 | L4 L9 L21 L22 L23 makes body 8 in component "BottomLeftCorner"
chamfer "Chamfer1''''''" distance 3 angle 45 2 edges at (-57.5, -62.5, 4) (-45, -75, 4) on bodies 8 in component "BottomLeftCorner"
sketch "Sketch1 (9)" plane through (0, 0, 0) normal (0, 0, 1) x (1, 0, 0) in component "TopLeftCorner"
  line L0 (-32.5, 71) -> (-32.5, 46)
  line L1 (-32.5, 62) -> (-28.5, 66)
  line L2 (-28.5, 71) -> (-28.5, 46)
  line L3 (-32.5, 55) -> (-28.5, 51)
  line L4 (-32.5, 46) -> (-57.5, 46)
  line L5 (-37.5, 50) -> (-41.5, 46)
  line L6 (-37.5, 50) -> (-52.5, 50)
  line L7 (-52.5, 50) -> (-48.5, 46)
  line L8 (-57.5, 71) -> (-32.5, 71)
  line L9 (-32.5, 71) -> (-32.5, 46)
  line L10 (-32.5, 46) -> (-57.5, 46)
  line L11 (-57.5, 46) -> (-57.5, 71)
  line L12 (-57.5, 46) -> (-48.5, 46)
  line L13 (-48.5, 46) -> (-52.5, 50)
  line L14 (-52.5, 50) -> (-37.5, 50)
  line L15 (-37.5, 50) -> (-41.5, 46)
  line L16 (-41.5, 46) -> (-32.5, 46)
  line L17 (-32.5, 55) -> (-28.5, 51)
  line L18 (-28.5, 51) -> (-28.5, 66)
  line L19 (-28.5, 66) -> (-32.5, 62)
  line L20 (-32.5, 55.1414) -> (-28.5, 51.1414)
  line L21 (-32.5, 61.8586) -> (-28.5, 65.8586)
  line L22 (-28.6, 65.7586) -> (-28.6, 51.2414)
  dimension "d201" = 0.1
  dimension "d202" = 0.1
  dimension "d203" = 0.1
  constraint horizontal L8
  constraint vertical L9
  constraint horizontal L10
  constraint vertical L11
  constraint coincident L0.end L4.start
  constraint coincident L0.start L8
  constraint coincident L4.end L11
  constraint coincident L4.end L10.end
  constraint coincident L7.end L12.end
  constraint coincident L6.end L7.start
  constraint coincident L5.start L6.start
  constraint coincident L5.end L15.end
  constraint coincident L3.start L17.start
  constraint coincident L3.end L17.end
  constraint coincident L1.end L18.end
  constraint coincident L1.start L19.end
  constraint coincident L9 L20.start
  constraint coincident L2 L20.end
  constraint coincident L9 L21.start
  constraint coincident L18 L21.end
  constraint coincident L21 L22.start
  constraint coincident L20 L22.end
  constraint parallel L2 L22
  constraint parallel L19 L21
  constraint parallel L17 L20
  measures "d201" distance of L19 L21
  measures "d202" distance of L17 L20
  measures "d203" distance of L2 L22
extrude "Extrude1''''''''" add sketch "Sketch1 (9)" along normal blind 4 separate body contours L0 L4 L5 L6 L7 L8 L9 L10 L11 L12 L13 L14 L15 L16 | L0 L9 L20 L21 L22 makes body 9 in component "TopLeftCorner"
fillet "Fillet1''''''" radius 1 8 edges at (-48.5, 46, 2) (-52.5, 50, 2) (-37.5, 50, 2) (-41.5, 46, 2) (-32.5, 55.1414, 2) (-32.5, 61.8586, 2) (-28.6, 65.7586, 2) (-28.6, 51.2414, 2) on bodies 9 in component "TopLeftCorner"
chamfer "Chamfer1'''''''" distance 3 angle 45 2 edges at (-45, 71, 4) (-57.5, 58.5, 4) on bodies 9 in component "TopLeftCorner"
fillet "Fillet1'''''''" radius 1 8 edges at (-37.7414, -46.1, 2) (-41.6414, -50, 2) (-48.3586, -50, 2) (-52.2586, -46.1, 2) (-32.5, -59.1414, 2) (-28.6, -69.7586, 2) (-28.6, -55.2414, 2) (-32.5, -65.8586, 2) on bodies 8 in component "BottomLeftCorner"
fillet "Fillet4" radius 1 12 edges at (-32.5, -59, 2.25) (-28.5, -55, 2.25) (-28.5, -70, 2.25) (-32.5, -66, 2.25) (-15.8586, -50, 2.25) (15.8586, -50, 2.25) (19.7586, -46.1, 2) (28.5, -59.1414, 2.25) (32.4, -55.2414, 2.25) (32.4, -69.7586, 2.25) (28.5, -65.8586, 2.25) (-19.7586, -46.1, 2) on bodies 5 in component "BottomEdge"
extrude "Extrude4" cut sketch "Sketch1" along normal up to surface (9 mm away) contours A0 | A1 bodies 1 in component "JarBase"
component "JarBase" placed x (1, 0, 0) y (0, 1, 0) z (0, 0, 1) at (0, 0, 0)
component "TopEdge" placed x (1, 0, 0) y (0, 1, 0) z (0, 0, 1) at (0, 0, 0)
component "RIghtEdge" placed x (1, 0, 0) y (0, 1, 0) z (0, 0, 1) at (0, 0, 0)
component "TopRightCorner" placed x (1, 0, 0) y (0, 1, 0) z (0, 0, 1) at (0, 0, 0)
component "BottomEdge" placed x (1, 0, 0) y (0, 1, 0) z (0, 0, 1) at (0, 0, 0)
component "RightBottomCorner" placed x (1, 0, 0) y (0, 1, 0) z (0, 0, 1) at (0, 0, 0)
component "LeftEdge" placed x (1, 0, 0) y (0, 1, 0) z (0, 0, 1) at (0, 0, 0)
component "BottomLeftCorner" placed x (1, 0, 0) y (0, 1, 0) z (0, 0, 1) at (0, 0, 0)
component "TopLeftCorner" placed x (1, 0, 0) y (0, 1, 0) z (0, 0, 1) at (0, 0, 0)
